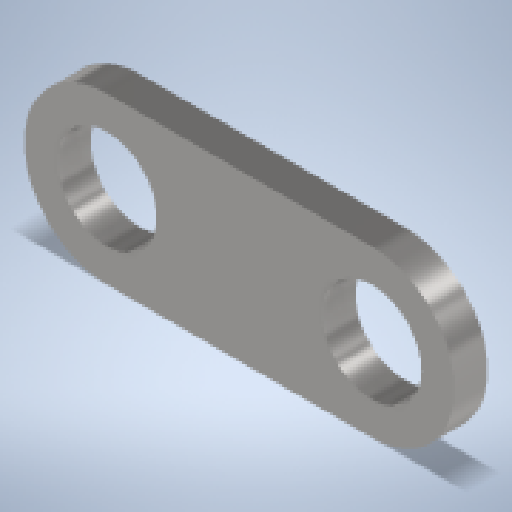
# Autodesk Inventor part: CompressionRollerActuatorLinkage1
Saved by Autodesk Inventor 2025 (Build 290162000, 162)
## iProperties
Created: 2024-08-19
Part Number: CompressionRollerActuatorLinkage1
Material: Stainless Steel
Document SubType Name: Modeling
Designer: hello
Density: 8 g/cm^3
Appearance: Semi-Polished
Author: hello
Autodesk Inventor part; units mm, degrees
ref_plane "YZ Plane" through (0, 0, 0) normal (1, 0, 0) x (0, 1, 0)
ref_plane "XZ Plane" through (0, 0, 0) normal (0, 1, 0) x (-1, 0, 0)
ref_plane "XY Plane" through (0, 0, 0) normal (0, 0, 1) x (1, 0, 0)
sketch "Sketch1" plane through (0, 0, 0) normal (0, 0, 1) x (1, 0, 0)
  line L0 (0, 0) -> (8, 0) construction
  line L1 (0, -2.5) -> (8, -2.5)
  line L2 (8, 2.5) -> (0, 2.5)
  arc A0 (0, 2.5) -> (0, -2.5) centre (0, 0) ccw
  arc A1 (8, -2.5) -> (8, 2.5) centre (8, 0) ccw
  circle A2 centre (8, 0) radius 1.5
  circle A3 centre (0, 0) radius 1.5
  point P0 (4, 0)
  dimension "d0" = 8
  dimension "d1" = 5
  dimension "d2" = 3
  dimension "d3" = 3
  constraints: 8 end point, 4 centre point, 4 point on circle, 4 tangent, 2 coincident, 1 horizontal, 1 midpoint, 1 parallel
  measures "d0" distance of L0.start L0.end
  measures "d1" diameter of A1
  measures "d2" diameter of A2
  measures "d3" diameter of A3
extrude "Extrusion1" add sketch "Sketch1" along normal mid plane 1
body "Solid1"
